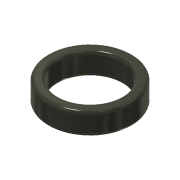
# Autodesk Inventor part: M16 - RX Coil
Saved by Autodesk Inventor 2016 (Build 200138000, 138)
## iProperties
Created: 2017-02-27
Part Number: M16 - RX Coil
Material: SAE 1020
Document SubType Name: Modeling
Designer: Fernando
Stock Number: 0
Mass: 326.724 g
Surface Area: 146.056 cm^2
Volume: 41.5151 cm^3
Density: 7.87 g/cm^3
Appearance: Gunmetal
SurfaceArea_m2: .01
Author: Fernando
Autodesk Inventor part; units mm, degrees
ref_plane "YZ Plane" through (0, 0, 0) normal (1, 0, 0) x (0, 1, 0)
ref_plane "XZ Plane" through (0, 0, 0) normal (0, 1, 0) x (-1, 0, 0)
ref_plane "XY Plane" through (0, 0, 0) normal (0, 0, 1) x (1, 0, 0)
sketch "Sketch2" plane through (0, 0, 0) normal (0, 0, 1) x (1, 0, 0)
  circle A0 centre (0, 0) radius 36
  circle A1 centre (0, 0) radius 43
  dimension "d16" = 86
  dimension "d17" = 72
  constraints: 2 centre point, 2 coincident
  measures "d16" diameter of A1
  measures "d17" diameter of A0
extrude "Extrusion2" add sketch "Sketch2" along normal blind 25
fillet "Fillet1" radius 3 4 edges at (-36, 0, 25) (-43, 0, 25) (-36, 0, 0) (-43, 0, 0)
body "Solid2"
